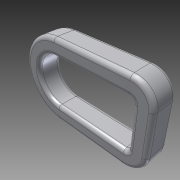
# Autodesk Inventor part: x_iddler_cap_zip_tie
Saved by Autodesk Inventor 2014 (Build 180170000, 170)
## iProperties
Created: 2014-03-25
Part Number: x_iddler_cap_zip_tie
Material: ABS Plastic
Document SubType Name: Modeling
Designer: buben
Density: 1.06 g/cm^3
Appearance: Smooth - White
Author: buben
Autodesk Inventor part; units mm, degrees
ref_plane "YZ Plane" through (0, 0, 0) normal (1, 0, 0) x (0, 1, 0)
ref_plane "XZ Plane" through (0, 0, 0) normal (0, 1, 0) x (-1, 0, 0)
ref_plane "XY Plane" through (0, 0, 0) normal (0, 0, 1) x (1, 0, 0)
sketch "Sketch1" plane through (0, 0, 0) normal (0, 1, 0) x (-1, 0, 0)
  line L0 (-9, -3) -> (0, -3)
  arc A0 (0, -3) -> (0, 3) centre (0, 0) ccw
  line L1 (0, 3) -> (-9, 3)
  arc A1 (-9.5, -2.5) -> (-9, -3) centre (-9, -2.5) ccw
  line L2 (-9.5, -2.5) -> (-9.5, 2.5)
  arc A2 (-9, 3) -> (-9.5, 2.5) centre (-9, 2.5) ccw
  line L3 (0, -5) -> (-9, -5)
  arc A3 (-11.5, -2.5) -> (-9, -5) centre (-9, -2.5) ccw
  line L4 (-11.5, -2.5) -> (-11.5, 2.5)
  arc A4 (-9, 5) -> (-11.5, 2.5) centre (-9, 2.5) ccw
  line L5 (-9, 5) -> (0, 5)
  arc A5 (0, -5) -> (0, 5) centre (0, 0) ccw
  dimension "d0" = 3
  dimension "d1" = 0.5
  dimension "d2" = 9.5
  dimension "d3" = 2
  constraints: 12 end point, 12 point on circle, 6 centre point, 6 tangent, 2 parallel, 2 perpendicular, 1 coincident, 1 horizontal, 1 vertical alignment, 5 other
  measures "d0" radius of A0
  measures "d1" radius of A1
  measures "d2" distance from line of L2 point (0, 0)
  measures "d3" distance between parallel lines of L4 L2
extrude "Extrusion1" add sketch "Sketch1" along normal blind 3
fillet "Fillet1" radius 0.5 24 edges at (10.7678, 3, 4.2678) (11.5, 3, 0) (10.7678, 3, -4.2678) (4.5, 3, -5) (-5, 3, 0) (4.5, 3, 5) (-3, 3, 0) (4.5, 3, -3) (9.3536, 3, -2.8536) (9.5, 3, 0) (9.3536, 3, 2.8536) (4.5, 3, 3) (-3, 0, 0) (4.5, 0, 3) (9.3536, 0, 2.8536) (9.5, 0, 0) (9.3536, 0, -2.8536) (4.5, 0, -3) (10.7678, 0, -4.2678) (11.5, 0, 0) (10.7678, 0, 4.2678) (4.5, 0, 5) (-5, 0, 0) (4.5, 0, -5)
body "Solid1"
